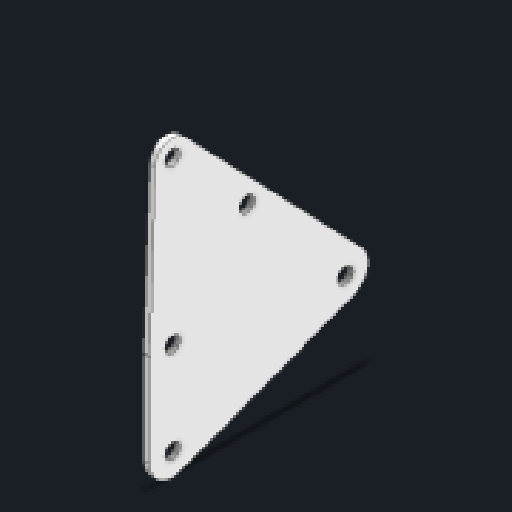
# Autodesk Inventor part: Gusset
Saved by Autodesk Inventor 2025.1 (Build 291241000, 241)
## iProperties
Created: 2024-11-28
Part Number: Gusset
Material: Acetal Resin, White
Document SubType Name: Modeling
Designer: avere
Density: 1.425 g/cm^3
Appearance: Smooth - White
Author: avere
Autodesk Inventor part; units mm, degrees
ref_plane "YZ Plane" through (0, 0, 0) normal (1, 0, 0) x (0, 1, 0)
ref_plane "XZ Plane" through (0, 0, 0) normal (0, 1, 0) x (-1, 0, 0)
ref_plane "XY Plane" through (0, 0, 0) normal (0, 0, 1) x (1, 0, 0)
sketch "Sketch1" plane through (0, 0, 0) normal (1, 0, 0) x (0, 1, 0)
  circle A0 centre (-29.9897, 25.7958) radius 2.1082
  circle A1 centre (-12.0119, -21.7167) radius 2.0955
  circle A2 centre (-4.5897, 25.7958) radius 2.0955
  arc A3 (-29.9897, 32.1458) -> (-35.9288, 23.5486) centre (-29.9897, 25.7958) ccw
  arc A4 (-17.951, -23.9639) -> (-7.6184, -26.3014) centre (-12.0119, -21.7167) ccw
  arc A5 (-4.3628, 32.1418) -> (-5.3835, 32.096) centre (-4.5897, 25.7958) ccw
  arc A6 (43.1561, 22.3566) -> (40.0311, 30.5545) centre (39.861, 25.7951) ccw
  line L0 (-29.9897, 32.1458) -> (-4.5897, 32.1458)
  line L1 (-35.9288, 23.5486) -> (-17.951, -23.9639)
  line L2 (-7.6184, -26.3014) -> (43.1561, 22.3566)
  line L3 (-4.3628, 32.1418) -> (40.0311, 30.5545)
  circle A7 centre (39.861, 25.7951) radius 2.1209
  circle A8 centre (18.5059, 5.3302) radius 2.0955
  point P0 (0, 0)
  dimension "d0" = 4.2164
  dimension "d1" = 4.191
  dimension "d2" = 12.7
  dimension "d3" = 12.7
  dimension "d4" = 12.7
  dimension "d5" = 9.525
  dimension "d6" = 4.2418
  dimension "d10" = 4.191
  constraints: 9 centre point, 9 point on circle, 8 end point, 7 tangent, 4 coincident, 2 other
  measures "d0" diameter of A0
  measures "d1" diameter of A1
  measures "d2" diameter of A3
  measures "d3" diameter of A4
  measures "d4" diameter of A5
  measures "d5" diameter of A6
  measures "d6" diameter of A7
  measures "d10" diameter of A8
extrude "Extrusion1" add sketch "Sketch1" along normal blind 1.5875
body "Solid1"
